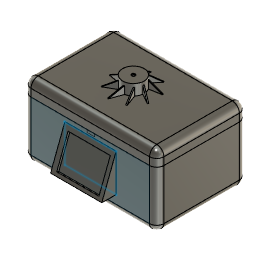
payload_v1 (Autodesk Fusion 360 design; units mm, degrees)
part number: 2026-08-17-00-12-50-066
Autodesk Fusion 360 part; units mm, degrees
sketch "Sketch1" plane through (0, 0, 0) normal (0, 0, 1) x (1, 0, 0)
  line L0 (-184.8982, 100.5485) -> (0, 100.5485)
  line L1 (0, 100.5485) -> (0, 0)
  line L2 (0, 0) -> (-184.8982, 0)
  line L3 (-184.8982, 0) -> (-184.8982, 100.5485)
  constraint horizontal L0
  constraint vertical L1
  constraint horizontal L2
  constraint vertical L3
  constraint coincident L1.end L2.start
extrude "Extrude1" add sketch "Sketch1" along normal blind 55 makes body 1
extrude "Extrude2" add 1 faces at (-61.6327, 33.5162, 55) along direction (0, 0, 1) blind 70 on bodies 1 bodies 1
fillet "Fillet1" radius 10 4 faces at (-61.6327, 33.5162, 125) (0, 67.0324, 41.6667) (-61.6327, 33.5162, 0) (-184.8982, 33.5162, 41.6667) on bodies 1
shell "Shell1" thickness 3 removed faces 0 bodies 1
move_body "Move1" bodies 1 to x (-1, 0, 0) y (0, 0, 1) z (0, 1, 0) at (-83.2188, 8.796, -6.2054)
ref_plane "WorkPlane1" through (9.2303, 71.296, 73.7946) normal (0, 0, -1) x (-1, 0, 0)
split "Split1" by plane through (9.2303, 71.296, 73.7946) normal (0, 0, -1) bodies 1 makes body 2 at (-18.2528, 53.796, -6.2054)
sketch "Sketch4" plane through (-80.2188, 0, 0) normal (1, 0, 0) x (0, 1, 0)
  line L0 (123.796, 73.7946) -> (18.796, 73.7946)
  line L1 (18.796, 73.7946) -> (18.796, 3.7946)
  line L2 (18.796, 3.7946) -> (123.796, 3.7946)
  line L3 (123.796, 3.7946) -> (123.796, 73.7946)
  circle A0 centre (80, 40) radius 24
  circle A1 centre (80, 40) radius 19
  dimension "d12" = 48
  dimension "d13" = 38
  constraint concentric A0 A1
  measures "d12" diameter of A0
  measures "d13" diameter of A1
extrude "Extrude3" add sketch "Sketch4" along normal blind 140 contours A0 bodies 2
sketch "Sketch5" plane through (-80.2188, 0, 0) normal (1, 0, 0) x (0, 1, 0)
  line L0 (123.796, 73.7946) -> (18.796, 73.7946)
  line L1 (18.796, 73.7946) -> (18.796, 3.7946)
  line L2 (18.796, 3.7946) -> (123.796, 3.7946)
  line L3 (123.796, 3.7946) -> (123.796, 73.7946)
  circle A0 centre (80, 40) radius 24
  circle A1 centre (35.8064, 47.1409) radius 16
  dimension "d16" = 32
  measures "d16" diameter of A1
extrude "Extrude4" add sketch "Sketch5" along normal blind 165 contours A1 bodies 2
ref_plane "WorkPlane2" through (9.2303, 71.296, 51.7946) normal (0, 0, 1) x (1, 0, 0)
sketch "Sketch7" plane through (-80.2188, 0, 0) normal (1, 0, 0) x (0, 1, 0)
  line L0 (123.796, 73.7946) -> (18.796, 73.7946)
  line L1 (18.796, 73.7946) -> (18.796, 3.7946)
  line L2 (18.796, 3.7946) -> (123.796, 3.7946)
  line L3 (123.796, 3.7946) -> (123.796, 73.7946)
  line L4 (21.0519, 53.3299) -> (52.8599, 53.3299)
  line L5 (52.8599, 53.3299) -> (52.8599, 70.0891)
  line L6 (52.8599, 70.0891) -> (21.0519, 70.0891)
  line L7 (21.0519, 70.0891) -> (21.0519, 53.3299)
  circle A0 centre (35.8064, 47.1409) radius 16
  circle A1 centre (80, 40) radius 24
  constraint horizontal L4
  constraint vertical L5
  constraint horizontal L6
  constraint vertical L7
  constraint coincident L4.start A0
extrude "Extrude5" cut sketch "Sketch7" along normal blind 165 contours L4 A0 | L4 L5 L6 L7 A0 picked at (38.0786, 56.092) bodies 2
sketch "Sketch8" plane through (-80.2188, 0, 0) normal (1, 0, 0) x (0, 1, 0)
  circle A0 centre (36.0552, 46.7697) radius 14
  dimension "d23" = 28
  measures "d23" diameter of A0
extrude "Extrude6" cut sketch "Sketch8" along normal blind 163 bodies 2
sketch "Sketch9" plane through (59.7812, 0, 0) normal (1, 0, 0) x (0, 1, 0)
  circle A0 centre (80, 40) radius 19
  circle A1 centre (80, 40) radius 24
  circle A2 centre (80, 40) radius 24
  circle A3 centre (80, 40) radius 5
  constraint concentric A0 A3
extrude "Extrude7" add sketch "Sketch9" along normal blind 3 contours A0 bodies 2
sketch "Sketch11" plane through (98.6794, 0, 0) normal (-1, 0, 0) x (0, -1, 0)
  line L0 (-18.796, 73.7946) -> (-123.796, 73.7946)
  line L1 (-123.796, 73.7946) -> (-123.796, 3.7946)
  line L2 (-123.796, 3.7946) -> (-18.796, 3.7946)
  line L3 (-18.796, 3.7946) -> (-18.796, 73.7946)
sketch "Sketch12" plane through (0, 0, 94.3432) normal (0, 0, 1) x (-1, 0, 0)
  line L0 (73.2188, -18.796) -> (-91.6794, -18.796)
  line L1 (-91.6794, -18.796) -> (-91.6794, -123.796)
  line L2 (-91.6794, -123.796) -> (73.2188, -123.796)
  line L3 (73.2188, -123.796) -> (73.2188, -18.796)
  circle A0 centre (-6.7055, -71.3462) radius 15
  dimension "d28" = 30
  measures "d28" diameter of A0
extrude "Extrude8" add sketch "Sketch12" along normal blind 15 contours A0 bodies 1
sketch "Sketch14" plane through (0, 0, 0) normal (1, 0, 0) x (0, 1, 0)
  line L0 (103.7018, 93.3906) -> (74.4371, 110.9684)
rib "Rib1" add thickness 1.5 on both sides direction (0, -0.514904, -0.857248) up to next extending the curves path "Sketch14" along L0 bodies 1
pattern_circular "C-Pattern1" count 9 over 360 about axis through (6.7055, 71.3462, 94.3432) along (0, 0, 1) of "Rib1"
hole "Hole1" at (6.7055, 71.3462, 109.3432) direction (0, 0, -1) diameter 3 depth 20 tip angle 180 counterbore diameter 5 counterbore depth 1 bodies 1
sketch "Sketch15" plane through (0, 8.796, 0) normal (0, -1, 0) x (1, 0, 0)
  line L0 (91.6794, 73.7946) -> (-73.2188, 73.7946)
  line L1 (-73.2188, 73.7946) -> (-73.2188, 3.7946)
  line L2 (-73.2188, 3.7946) -> (91.6794, 3.7946)
  line L3 (91.6794, 3.7946) -> (91.6794, 73.7946)
  line L4 (-26.054, 67.7879) -> (45.2264, 67.7879)
  line L5 (45.2264, 67.7879) -> (45.2264, 15.633)
  line L6 (45.2264, 15.633) -> (-26.054, 15.633)
  line L7 (-26.054, 15.633) -> (-26.054, 67.7879)
  constraint horizontal L4
  constraint vertical L5
  constraint horizontal L6
  constraint vertical L7
extrude "Extrude11" add sketch "Sketch15" along normal blind 20 contours L4 L5 L6 L7 bodies 2
sketch "Sketch18" plane through (-26.054, 0, 0) normal (-1, 0, 0) x (0, -1, 0)
  line L0 (-8.796, 67.7879) -> (-8.796, 15.633)
  line L1 (-8.796, 15.633) -> (11.204, 15.633)
  line L2 (11.204, 15.633) -> (11.204, 67.7879)
  line L3 (11.204, 67.7879) -> (-8.796, 67.7879)
  line L4 (-8.796, 67.7879) -> (11.204, 15.633)
  constraint coincident L0.start L3.end
  constraint coincident L1.end L2.start
extrude "Extrude12" cut sketch "Sketch18" against normal blind 64 contours L2 L3 L4 bodies 2
sketch "Sketch20" plane through (0, 11.796, 0) normal (0, 1, 0) x (-1, 0, 0)
  line L0 (73.2188, 73.7946) -> (-91.6794, 73.7946)
  line L1 (-91.6794, 73.7946) -> (-91.6794, 3.7946)
  line L2 (-91.6794, 3.7946) -> (73.2188, 3.7946)
  line L3 (73.2188, 3.7946) -> (73.2188, 73.7946)
  line L4 (17, 73) -> (35.556, 73)
  line L5 (35.556, 73) -> (35.556, 49.5)
  line L6 (35.556, 49.5) -> (17, 49.5)
  line L7 (17, 49.5) -> (17, 73)
  line L8 (34.056, 71.5) -> (34.056, 51)
  line L9 (34.056, 51) -> (18.5, 51)
  line L10 (18.5, 51) -> (18.5, 71.5)
  line L11 (18.5, 71.5) -> (34.056, 71.5)
  dimension "d52" = 23.5
  dimension "d57" = 1.5
  constraint horizontal L4
  constraint vertical L5
  constraint horizontal L6
  constraint vertical L7
  measures "d52" distance of L4.start L6.end
ref_plane "WorkPlane3" through (-26.278, 13.296, 61.25) normal (0, 1, 0) x (-1, 0, 0)
ref_plane "WorkPlane4" through (-26.278, 13.296, 61.25) normal (0, 1, 0) x (-1, 0, 0)
extrude "Extrude13" add sketch "Sketch20" along normal blind 3 contours L4 L5 L6 L7 bodies 2
sketch "Sketch21" plane through (0, 14.796, 0) normal (0, 1, 0) x (-1, 0, 0)
  line L0 (18.5, 51) -> (18.5, 71.5)
  line L1 (18.5, 71.5) -> (34.056, 71.5)
  line L2 (34.056, 71.5) -> (34.056, 51)
  line L3 (34.056, 51) -> (18.5, 51)
  line L4 (17, 49.5) -> (35.556, 49.5)
  line L5 (35.556, 49.5) -> (35.556, 73)
  line L6 (35.556, 73) -> (17, 73)
  line L7 (17, 73) -> (17, 49.5)
  line L8 (17, 71) -> (35.556, 71)
  line L9 (35.556, 71) -> (35.556, 51.1682)
  line L10 (35.556, 51.1682) -> (17, 51.1682)
  line L11 (17, 51.1682) -> (17, 71)
  constraint horizontal L8
  constraint vertical L9
  constraint horizontal L10
  constraint vertical L11
  constraint coincident L5 L9.end
  constraint coincident L7 L8.start
extrude "Extrude14" cut sketch "Sketch21" against normal blind 3 contours L0 L7 L8 L10 L11 bodies 2
extrude "Extrude15" cut sketch "Sketch21" against normal blind 3 contours L2 L5 L8 L9 L10 bodies 2
sketch "Sketch22" plane through (0, -14.9939, 5.7498) normal (0, -0.933702, 0.35805) x (1, 0, 0)
  line L0 (37.946, 66.4431) -> (-26.054, 66.4431)
  line L1 (-26.054, 66.4431) -> (-26.054, 10.585)
  line L2 (-26.054, 10.585) -> (37.946, 10.585)
  line L3 (37.946, 10.585) -> (37.946, 66.4431)
extrude "Extrude16" cut sketch "Sketch18" along normal blind 0 and the other way blind 100 contours L2 L3 L4 bodies 2
sketch "Sketch23" plane through (0, -14.9939, 5.7498) normal (0, -0.933702, 0.35805) x (1, 0, 0)
  line L0 (-26.054, 66.4431) -> (-26.054, 10.585)
  line L1 (-26.054, 10.585) -> (45.2264, 10.585)
  line L2 (45.2264, 10.585) -> (45.2264, 66.4431)
  line L3 (45.2264, 66.4431) -> (-26.054, 66.4431)
  line L4 (-19.0726, 59.295) -> (39.6557, 59.295)
  line L5 (39.6557, 59.295) -> (39.6557, 15.295)
  line L6 (39.6557, 15.295) -> (-19.0726, 15.295)
  line L7 (-19.0726, 15.295) -> (-19.0726, 59.295)
  dimension "d68" = 44
  constraint horizontal L4
  constraint vertical L5
  constraint horizontal L6
  constraint vertical L7
  measures "d68" distance of L4.start L6.end
extrude "Extrude17" cut sketch "Sketch23" against normal blind 3 contours L4 L5 L6 L7 bodies 2
sketch "Sketch24" plane through (0, 0, 73.7946) normal (0, 0, 1) x (-1, 0, 0)
  arc A0 (80.2188, -18.796) -> (73.2188, -11.796) centre (73.2188, -18.796) ccw
  line L0 (80.2188, -18.796) -> (80.2188, -123.796)
  arc A1 (73.2188, -130.796) -> (80.2188, -123.796) centre (73.2188, -123.796) ccw
  line L1 (73.2188, -130.796) -> (-91.6794, -130.796)
  arc A2 (-98.6794, -123.796) -> (-91.6794, -130.796) centre (-91.6794, -123.796) ccw
  line L2 (-98.6794, -123.796) -> (-98.6794, -18.796)
  arc A3 (-91.6794, -11.796) -> (-98.6794, -18.796) centre (-91.6794, -18.796) ccw
  line L3 (-91.6794, -11.796) -> (73.2188, -11.796)
  arc A4 (83.2188, -18.796) -> (73.2188, -8.796) centre (73.2188, -18.796) ccw
  line L4 (73.2188, -8.796) -> (-91.6794, -8.796)
  arc A5 (-91.6794, -8.796) -> (-101.6794, -18.796) centre (-91.6794, -18.796) ccw
  line L5 (-101.6794, -18.796) -> (-101.6794, -123.796)
  arc A6 (-101.6794, -123.796) -> (-91.6794, -133.796) centre (-91.6794, -123.796) ccw
  line L6 (-91.6794, -133.796) -> (73.2188, -133.796)
  arc A7 (73.2188, -133.796) -> (83.2188, -123.796) centre (73.2188, -123.796) ccw
  line L7 (83.2188, -123.796) -> (83.2188, -18.796)
  line L8 (-15, -9.5) -> (-4.5, -9.5)
  line L9 (-4.5, -9.5) -> (-4.5, -11.5)
  line L10 (-4.5, -11.5) -> (-15, -11.5)
  line L11 (-15, -11.5) -> (-15, -9.5)
  constraint horizontal L8
  constraint vertical L9
  constraint horizontal L10
  constraint vertical L11
extrude "Extrude18" cut sketch "Sketch24" against normal blind 4 contours L8 L9 L10 L11 bodies 2
